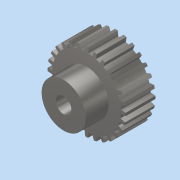
# Autodesk Inventor part: largeIdlerPinion
Saved by Autodesk Inventor 2017 (Build 210142000, 142)
## iProperties
Created: 2016-11-30
Part Number: largeIdlerPinion
Material: Steel, Carbon
Document SubType Name: Modeling
Designer: techn
Density: 7.85 g/cm^3
Appearance: Semi-Polished
Author: techn
Comments: A pinion gear i already own of the 20 to 24 tooth variety - adjust mesh in ballast section based on the axle pitch
Autodesk Inventor part; units mm, degrees
ref_plane "YZ Plane" through (0, 0, 0) normal (1, 0, 0) x (0, 1, 0)
ref_plane "XZ Plane" through (0, 0, 0) normal (0, 1, 0) x (-1, 0, 0)
ref_plane "XY Plane" through (0, 0, 0) normal (0, 0, 1) x (1, 0, 0)
sketch "Sketch1" plane through (0, 0, 0) normal (0, 0, 1) x (1, 0, 0)
  circle A0 centre (0, 0) radius 7.0358
  dimension "d0" = 14.0716
  constraints: 1 centre point, 1 coincident
  measures "d0" diameter of A0
extrude "Extrusion1" add sketch "Sketch1" along normal blind 6.096
sketch "Sketch2" plane through (0, 0, 6.096) normal (0, 0, 1) x (1, 0, 0)
  circle A0 centre (0, 0) radius 4.5085
  dimension "d3" = 9.017
  constraints: 1 centre point, 1 coincident
  measures "d3" diameter of A0
extrude "Extrusion2" add sketch "Sketch2" along normal blind 4.699
sketch "Sketch3" plane through (0, 0, 10.795) normal (0, 0, 1) x (1, 0, 0)
  circle A0 centre (0, 0) radius 1.5875
  dimension "d6" = 3.175
  constraints: 1 centre point, 1 coincident
  measures "d6" diameter of A0
extrude "Extrusion3" cut sketch "Sketch3" against normal blind 25.4
sketch "Sketch5" plane through (0, 0, 0) normal (0, 0, -1) x (-1, 0, 0)
  line L0 (-0.3683, 7.0262) -> (0.3683, 7.0262)
  line L1 (0.3683, 7.0262) -> (0.3683, 7.4072)
  line L2 (0.3683, 7.4072) -> (0.2921, 7.9914)
  line L3 (0.2921, 7.9914) -> (-0.2921, 7.9914)
  line L4 (-0.2921, 7.9914) -> (-0.3683, 7.4072)
  line L5 (-0.3683, 7.4072) -> (-0.3683, 7.0262)
  circle A0 centre (0, 0) radius 7.0358 projected
  point P0 (0, 7.9914)
  point P1 (0, 7.0262)
  dimension "d20" = 0.5842
  dimension "d21" = 0.7366
  dimension "d22" = 0.381
  dimension "d23" = 0.5842
  constraints: 12 end point, 2 midpoint, 2 parallel, 2 vertical alignment, 1 horizontal, 1 horizontal alignment, 1 perpendicular, 2 other
  measures "d20" distance of L2.end L3.end
  measures "d21" distance of L0.start L0.end
  measures "d22" distance of L0.end L1.end
  measures "d23" distance from line of L4.end L3
extrude "Extrusion5" add sketch "Sketch5" against normal up to surface (6.096 mm away) contours A0 L0 | L5 L4 L3 L2 L1 A0 picked at (-0.0409, 7.029)
pattern_circular "Circular Pattern1" count 28 over 360 about axis through (0, 0, 0) along (0, 0, 1) of "Extrusion5"
body "Solid1"
